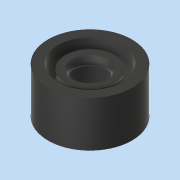
# Autodesk Inventor part: RubberMould
Saved by Autodesk Inventor 2017 (Build 210142000, 142)
## iProperties
Created: 2016-10-13
Part Number: RubberMould
Material: Generic
Document SubType Name: Modeling
Designer: techn
Density: 1 g/cm^3
Appearance: Smooth - Black
Author: techn
Autodesk Inventor part; units mm, degrees
ref_plane "YZ Plane" through (0, 0, 0) normal (1, 0, 0) x (0, 1, 0)
ref_plane "XZ Plane" through (0, 0, 0) normal (0, 1, 0) x (-1, 0, 0)
ref_plane "XY Plane" through (0, 0, 0) normal (0, 0, 1) x (1, 0, 0)
sketch "Sketch1" plane through (0, 0, 0) normal (0, 0, 1) x (1, 0, 0)
  line L0 (0, 0) -> (5.5, 0)
  line L1 (5.5, 0) -> (5.5, 6)
  line L2 (5.5, 6) -> (4.23, 6)
  line L3 (4.23, 6) -> (4.23, 1.555)
  line L4 (0, 4.7594) -> (2, 4.7594)
  line L5 (4.23, 1.555) -> (2.96, 1.555)
  line L6 (2, 4.7594) -> (2, 4.1244)
  line L7 (2, 4.1244) -> (2.3175, 4.1244)
  arc A0 (2.3175, 5.3944) -> (2.3175, 4.1244) centre (2.7937, 4.7594) ccw
  line L8 (2.3175, 4.1244) -> (2.96, 1.555)
  line L9 (2.3175, 5.3944) -> (3.2065, 5.3944)
  arc A1 (3.2065, 5.3944) -> (3.2065, 4.1244) centre (3.9012, 4.7594) ccw
  line L10 (3.2065, 4.1244) -> (3.849, 1.555)
  line L11 (2.96, 1.555) -> (2.96, 0)
  line L12 (0, 0) -> (0, 3.2708)
  dimension "d0" = 5.5
  dimension "d1" = 6
  dimension "d2" = 1.27
  dimension "d3" = 4.445
  dimension "d4" = 2
  dimension "d5" = 1.27
  dimension "d6" = 0.635
  dimension "d7" = 0.3175
  dimension "d8" = 1.27
  dimension "d9" = 0.889
  constraints: 26 end point, 6 horizontal, 5 point on circle, 3 perpendicular, 2 centre point, 2 point on line, 2 vertical
  measures "d0" distance of L0.start L0.end
  measures "d1" distance of L0.end L1.end
  measures "d2" distance of L1.end L2.end
  measures "d3" distance of L2.end L3.end
  measures "d4" distance of L4.start L4.end
  measures "d5" distance of L3.end L5.end
  measures "d6" distance of L4.end L6.end
  measures "d7" distance of L6.end L7.end
  measures "d8" distance of L7.end L9.start
  measures "d9" distance of L9.start L9.end
revolve "Revolution1" add sketch "Sketch1" angle 360 about axis through (0, 0, 0) along (0, 1, 0) contours L11 L5 L3 L2 L1 L0 | L8 A0 L9 A1 L10 L5
body "Solid1"
